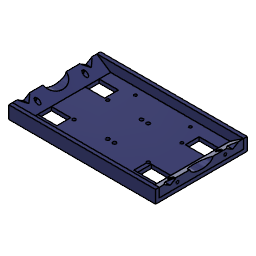
Techo 1 (Autodesk Fusion 360 design; units mm, degrees)
Autodesk Fusion 360 part; units mm, degrees
note: some values were not read from the file. Set by a fixed rule: which sketch regions a step uses.
sketch "Boceto1" plane through (0, 0, 0) normal (0, 1, 0) x (1, 0, 0)
  line L0 (-50, 25) -> (110, 25)
  line L1 (110, 25) -> (110, -75)
  line L2 (110, -75) -> (-50, -75)
  line L3 (-50, -75) -> (-50, 25)
  dimension "d1" = 160
  dimension "d2" = 100
  constraint horizontal L0
  constraint perpendicular L0 L1
  constraint perpendicular L1 L2
  constraint perpendicular L0 L3
  measures "d1" distance of L0.start L0.end
  measures "d2" distance of L0.end L1.end
extrude "Extruir1" add sketch "Boceto1" along normal blind 4 makes body 1
sketch "Boceto2" plane through (0, 4, 0) normal (0, 1, 0) x (-1, 0, 0)
  line L0 (50, 75) -> (-110, 75)
  line L1 (-110, 75) -> (-110, -25)
  line L2 (-110, -25) -> (50, -25)
  line L3 (50, -25) -> (50, 75)
  line L4 (50, -25) -> (50, -21)
  line L5 (50, -21) -> (-110, -21)
  line L6 (-110, -25) -> (50, -25)
  line L7 (50, 75) -> (50, 71)
  line L8 (-110, 75) -> (50, 75)
  line L9 (-110, 75) -> (-110, 71)
  line L10 (50, 71) -> (-110, 71)
  dimension "d5" = 4
  dimension "d6" = 4
  dimension "d14" = 4
  constraint coincident L2.end L3.start
  constraint perpendicular L2 L4
  constraint coincident L1 L5.end
  constraint perpendicular L1 L5
  constraint coincident L1.end L2.start
  constraint coincident L0.start L3.end
  constraint perpendicular L0 L7
  constraint coincident L0.end L1.start
  constraint perpendicular L8 L9
  measures "d5" distance of L2.end L4.end
  measures "d6" distance of L0.start L7.end
  measures "d14" distance of L0.end L9.end
extrude "Extruir2" add sketch "Boceto2" along normal blind 10 contours L0 L1 L3 L7 L8 L9 L10 | L1 L2 L3 L4 L5 L6 bodies 1
sketch "Boceto3" plane through (0, 4, 0) normal (0, 1, 0) x (-1, 0, 0)
  line L0 (-110, 71) -> (-110, -21)
  line L1 (-110, -21) -> (50, -21)
  line L2 (50, -21) -> (50, 71)
  line L3 (50, 71) -> (-110, 71)
sketch "Boceto4" plane through (0, 0, -21) normal (0, 0, 1) x (1, 0, 0)
  line L0 (-50, 4) -> (110, 4)
  line L1 (110, 4) -> (110, 14)
  line L2 (110, 14) -> (-50, 14)
  line L3 (-50, 14) -> (-50, 4)
  line L4 (-50, 0) -> (-50, 4)
  line L5 (-50, 4) -> (-50, 14)
  line L6 (-50, 4) -> (-35, 4)
  line L7 (-50, 14) -> (-35, 4)
  line L8 (110, 4) -> (95, 4)
  line L9 (110, 4) -> (110, 14)
  line L10 (110, 14) -> (95, 4)
  dimension "d9" = 10
  dimension "d10" = 15
  dimension "d11" = 10
  constraint coincident L0.start L3.end
  constraint perpendicular L0 L4
  constraint perpendicular L2 L5
  constraint coincident L0 L6.end
  constraint coincident L0.end L1.start
  constraint perpendicular L1 L8
  constraint perpendicular L0 L9
  measures "d9" distance of L0.start L2.end
  measures "d10" distance of L0.end L8.end
  measures "d11" distance of L0.end L1.end
extrude "Extruir3" add sketch "Boceto4" along normal blind 92 separate body contours L0 L3 L5 L6 L7 | L0 L1 L8 L9 L10 makes body 2 at (-45, 10.6667, 9.6667) makes body 3 at (105, 10.6667, 9.6667)
sketch "Boceto6" plane through (0, 0, 71) normal (0, 0, -1) x (-1, 0, 0)
  line L0 (-110, 4) -> (50, 4)
  line L1 (50, 4) -> (50, 14)
  line L2 (50, 14) -> (-110, 14)
  line L3 (-110, 14) -> (-110, 4)
  line L4 (-110, 4) -> (-106, 4)
  line L5 (-106, 4) -> (-106, 9)
  line L6 (-110, 4) -> (-106, 4)
  line L7 (-106, 4) -> (-91, 4)
  line L8 (-91, 4) -> (-91, 9)
  line L9 (-91, 4) -> (-91, 9)
  dimension "d15" = 5
  constraint coincident L0.start L3.end
  constraint coincident L0 L4.end
  constraint perpendicular L0 L5
  constraint coincident L0 L7.end
  constraint perpendicular L7 L8
  measures "d15" distance of L4.end L5.end
sketch "Boceto7" plane through (0, 0, 0) normal (1, 0, 0) x (0, 0, -1)
  line L0 (-71, 4) -> (-71, 9)
  line L1 (-71, 9) -> (-69, 9)
  line L2 (-69, 9) -> (-51, 9)
  circle A0 centre (-51, 9) radius 2
  line L3 (-51, 9) -> (1, 9)
  circle A1 centre (1, 9) radius 2
  dimension "d16" = 2
  dimension "d17" = 18
  dimension "d22" = 4
  dimension "d31" = 52
  dimension "d32" = 4
  constraint vertical L0
  constraint perpendicular L0 L1
  constraint perpendicular L0 L2
  constraint coincident L2.end A0.centre
  constraint parallel L2 L3
  constraint coincident L3.end A1.centre
  measures "d16" distance of L0.end L1.end
  measures "d17" distance of L1.end L2.end
  measures "d22" diameter of A0
  measures "d31" distance of L2.end L3.end
  measures "d32" diameter of A1
extrude "Extruir4" cut sketch "Boceto7" along normal blind 104 contours L2 A0 L3 | L2 A0 L3 bodies 3
extrude "Extruir5" cut sketch "Boceto7" against normal blind 45.5 contours L2 A0 L3 | L2 A0 L3 bodies 2
sketch "Boceto9" plane through (-50, 0, 0) normal (-1, 0, 0) x (0, 0, 1)
  line L0 (-25, 0) -> (75, 0)
  line L1 (75, 0) -> (75, 14)
  line L2 (75, 14) -> (71, 14)
  line L3 (71, 14) -> (71, 4)
  line L4 (71, 4) -> (-21, 4)
  line L5 (-21, 4) -> (-21, 14)
  line L6 (-21, 14) -> (-25, 14)
  line L7 (-25, 14) -> (-25, 0)
  circle A0 centre (-1, 9) radius 1.5
  circle A1 centre (51, 9) radius 1.5
  dimension "d25" = 3
  dimension "d26" = 3
  measures "d25" diameter of A0
  measures "d26" diameter of A1
extrude "Extruir6" cut sketch "Boceto9" along normal mid plane 394 contours A0 | A1 bodies 3
extrude "Extruir8" cut sketch "Boceto7" against normal blind 45.5 contours A1 bodies 2
extrude "Extruir9" cut sketch "Boceto7" along normal blind 105.5 contours A1 bodies 3
extrude "Extruir7" cut sketch "Boceto9" against normal blind 56 contours A0 | A1 bodies 2
sketch "Boceto11" plane through (0, 4, 0) normal (0, 1, 0) x (-1, 0, 0)
  line L0 (50, 71) -> (-110, 71)
  line L1 (-110, 71) -> (-110, -21)
  line L2 (-110, -21) -> (50, -21)
  line L3 (50, -21) -> (50, 71)
  line L4 (-30, -21) -> (-30, 25)
  line L5 (-30, -21) -> (25, -21)
  line L6 (34, -25) -> (34, -1)
  line L7 (34, -1) -> (14, -1)
  line L8 (14, -1) -> (14, -8.5)
  line L9 (14, -8.5) -> (35, -8.5)
  line L10 (35, -8.5) -> (35, 6.5)
  line L11 (35, 6.5) -> (14, 6.5)
  line L12 (14, 6.5) -> (14, -1)
  line L13 (35, 75) -> (35, 51)
  line L14 (35, 51) -> (35, 43.5)
  line L15 (35, 43.5) -> (14, 43.5)
  line L16 (14, 43.5) -> (14, 58.5)
  line L17 (14, 58.5) -> (35, 58.5)
  line L18 (-90, 75) -> (-90, 51)
  line L19 (-90, 51) -> (-91, 51)
  line L20 (-91, 51) -> (-91, 43.5)
  line L21 (-91, 43.5) -> (-70, 43.5)
  line L22 (-70, 43.5) -> (-70, 58.5)
  line L23 (-70, 58.5) -> (-91, 58.5)
  line L24 (-91, 58.5) -> (-91, 51)
  line L25 (-91, -25) -> (-91, -1)
  line L26 (-91, -1) -> (-91, 6.5)
  line L27 (-91, 6.5) -> (-70, 6.5)
  line L28 (-70, 6.5) -> (-70, -8.5)
  line L29 (-70, -8.5) -> (-91, -8.5)
  line L30 (-41.25, -11.4952) -> (-30, -17.9904)
  line L31 (-30, -17.9904) -> (-18.75, -11.4952)
  line L32 (-91, -8.5) -> (-95, -8.5)
  line L33 (-95, -8.5) -> (-95, 6.5)
  line L34 (-91, 6.5) -> (-95, 6.5)
  line L35 (-91, 43.5) -> (-95, 43.5)
  line L36 (-95, 43.5) -> (-95, 58.5)
  line L37 (-95, 58.5) -> (-91, 58.5)
  line L38 (-70, 43.5) -> (-74, 43.5)
  line L39 (-74, 43.5) -> (-74, 58.5)
  dimension "d49" = 24
  dimension "d50" = 20
  dimension "d51" = 7.5
  dimension "d52" = 15
  dimension "d54" = 24
  dimension "d55" = 7.5
  dimension "d56" = 21
  dimension "d57" = 15
  dimension "d58" = 24
  dimension "d59" = 7.5
  dimension "d60" = 21
  dimension "d61" = 15
  dimension "d62" = 24
  dimension "d63" = 7.5
  dimension "d64" = 21
  dimension "d65" = 15
  dimension "d89" = 4
  constraint midpoint L2 L4.start
  constraint perpendicular L2 L4
  constraint coincident L2 L5.end
  constraint vertical L6
  constraint perpendicular L6 L7
  constraint perpendicular L7 L8
  constraint perpendicular L6 L9
  constraint perpendicular L9 L10
  constraint perpendicular L8 L11
  constraint perpendicular L7 L12
  constraint perpendicular L0 L13
  constraint perpendicular L0 L14
  constraint perpendicular L3 L15
  constraint perpendicular L0 L16
  constraint coincident L13 L17.end
  constraint perpendicular L13 L17
  constraint perpendicular L0 L18
  constraint perpendicular L18 L19
  constraint perpendicular L19 L20
  constraint perpendicular L20 L21
  constraint perpendicular L21 L22
  constraint perpendicular L18 L23
  constraint perpendicular L19 L24
  constraint perpendicular L2 L25
  constraint perpendicular L2 L26
  constraint perpendicular L26 L27
  constraint perpendicular L27 L28
  constraint coincident L25 L29.end
  constraint perpendicular L25 L29
  constraint perpendicular L25 L32
  constraint perpendicular L27 L33
  constraint perpendicular L33 L34
  constraint perpendicular L20 L35
  constraint perpendicular L23 L36
  constraint perpendicular L24 L37
  constraint perpendicular L22 L38
  constraint perpendicular L21 L39
  measures "d49" distance of L6.start L6.end
  measures "d50" distance of L6.end L7.end
  measures "d51" distance of L7.end L8.end
  measures "d52" distance of L9.end L10.end
  measures "d54" distance of L13.start L13.end
  measures "d55" distance of L13.end L14.end
  measures "d56" distance of L14.end L15.end
  measures "d57" distance of L15.end L16.end
  measures "d58" distance of L18.start L18.end
  measures "d59" distance of L19.end L20.end
  measures "d60" distance of L20.end L21.end
  measures "d61" distance of L21.end L22.end
  measures "d62" distance of L25.start L25.end
  measures "d63" distance of L25.end L26.end
  measures "d64" distance of L26.end L27.end
  measures "d65" distance of L27.end L28.end
  measures "d89" distance of L21.end L38.end
extrude "Extruir12" cut sketch "Boceto11" against normal blind 14 contours L6 L7 L8 L9 | L6 L7 L9 L10 L11 L12 | L13 L14 L15 L16 L17 | L18 L19 L20 L21 L23 L39 | L18 L19 L23 L24 | L21 L22 L23 L38 L39 | L25 L26 L27 L28 L29 bodies 1
sketch "Boceto12" plane through (-50, 0, 0) normal (-1, 0, 0) x (0, 0, 1)
  circle A0 centre (-1, 9) radius 1.5
  circle A1 centre (51, 9) radius 1.5
  line L0 (-21, 14) -> (-21, 4)
  line L1 (-21, 4) -> (71, 4)
  line L2 (71, 4) -> (71, 14)
  line L3 (71, 14) -> (-21, 14)
  line L4 (-9, 10) -> (-15.0622, 13.5)
  line L5 (-15.0622, 13.5) -> (-15.0622, 20.5)
  line L6 (-15.0622, 20.5) -> (-9, 24)
  line L7 (-9, 24) -> (-2.9378, 20.5)
  line L8 (-2.9378, 20.5) -> (-2.9378, 13.5)
  line L9 (-2.9378, 13.5) -> (-9, 10)
  ellipse E0 centre (25, 14) end of major axis (37.5, 14) minor radius 6
  line L10 (65.0622, 13.5) -> (59, 10)
  line L11 (59, 10) -> (52.9378, 13.5)
  line L12 (52.9378, 13.5) -> (52.9378, 20.5)
  line L13 (65.0622, 20.5) -> (65.0622, 13.5)
  line L14 (59, 24) -> (65.0622, 20.5)
  line L15 (52.9378, 20.5) -> (59, 24)
extrude "Extruir13" cut sketch "Boceto12" against normal blind 186 contours L3 L4 L5 L8 L9 | L3 E0 | L3 L10 L11 L12 L13 picked at (25.1662, 12.0016) bodies 2 3
extrude "Extruir14" cut sketch "Boceto7" along normal blind 105.5 contours L2 A0 L3 | L2 A0 L3 bodies 3
extrude "Extruir15" cut sketch "Boceto11" against normal blind 15 contours L20 L24 L35 L36 L37 | L25 L26 L32 L33 L34 bodies 1
extrude "Extruir16" add sketch "Boceto11" against normal blind 4 separate body contours L21 L22 L23 L38 L39 makes body 4
sketch "Boceto13" plane through (0, 4, 0) normal (0, 1, 0) x (-1, 0, 0)
  line L0 (-70, -8.5) -> (-74, -8.5)
  line L1 (-74, -8.5) -> (-74.1, 6.5)
  line L2 (-74.1, 6.5) -> (-70, 6.5)
  line L3 (-70, 6.5) -> (-70, -8.5)
  dimension "d94" = 4
  constraint horizontal L0
  constraint parallel L0 L2
  measures "d94" distance of L0.start L0.end
extrude "Extruir17" add sketch "Boceto13" against normal blind 4 bodies 1
sketch "Boceto15" plane through (0, 4, 0) normal (0, 1, 0) x (-1, 0, 0)
  line L0 (50, 71) -> (-110, 71)
  line L1 (-110, 71) -> (-110, -21)
  line L2 (-110, -21) -> (50, -21)
  line L3 (50, -21) -> (50, 71)
  line L4 (35, -8.5) -> (14, -8.5)
  line L5 (14, -8.5) -> (14, 6.5)
  line L6 (14, 6.5) -> (35, 6.5)
  line L7 (35, 6.5) -> (35, -8.5)
  line L8 (-70, 43.5) -> (-95, 43.5)
  line L9 (-95, 43.5) -> (-95, 58.5)
  line L10 (-95, 58.5) -> (-70, 58.5)
  line L11 (-70, 58.5) -> (-70, 43.5)
  line L12 (35, 43.5) -> (14, 43.5)
  line L13 (14, 43.5) -> (14, 58.5)
  line L14 (14, 58.5) -> (35, 58.5)
  line L15 (35, 58.5) -> (35, 43.5)
  line L16 (-95, 6.5) -> (-74.1, 6.5)
  line L17 (-74.1, 6.5) -> (-74, -8.5)
  line L18 (-74, -8.5) -> (-95, -8.5)
  line L19 (-95, -8.5) -> (-95, 6.5)
  circle A0 centre (-70.35, 43.35) radius 1.7
  circle A1 centre (10.35, 43.35) radius 1.7
  circle A2 centre (0, 63) radius 1.5
  circle A3 centre (-26.35, 43.35) radius 1.85
  circle A4 centre (-33.65, 43.35) radius 1.85
  circle A5 centre (-60, 63) radius 1.5
  circle A6 centre (-33.65, 6.65) radius 1.85
  circle A7 centre (-26.35, 6.65) radius 1.85
  circle A8 centre (10.35, 6.65) radius 1.7
  circle A9 centre (0, -13) radius 1.5
  circle A10 centre (-60, -13) radius 1.5
  circle A11 centre (-70.35, 6.65) radius 1.55
  point P0 (-35.5, 6.65)
extrude "Extruir19" cut sketch "Boceto15" against normal blind 40 contours L8 L11 A0 | L8 L11 A0 | A1 | A2 | A3 | A4 | A5 | A6 | A7 | A8 | A9 | A10 | A11 bodies 1 4
